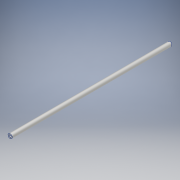
# Autodesk Inventor part: ScrewDriver
Saved by Autodesk Inventor 2017 (Build 210142000, 142)
## iProperties
Created: 2016-11-27
Part Number: ScrewDriver
Material: Aluminum 6061
Document SubType Name: Modeling
Designer: umr
Density: 2.7 g/cm^3
Appearance: Aluminum - Flat
Author: umr
Autodesk Inventor part; units mm, degrees
ref_plane "YZ Plane" through (0, 0, 0) normal (1, 0, 0) x (0, 1, 0)
ref_plane "XZ Plane" through (0, 0, 0) normal (0, 1, 0) x (-1, 0, 0)
sketch "Sketch1" plane through (0, 0, 0) normal (0, 1, 0) x (-1, 0, 0)
  circle A0 centre (0, 0) radius 8
  dimension "d0" = 16
  constraints: 1 centre point, 1 coincident
  measures "d0" diameter of A0
extrude "Extrusion1" add sketch "Sketch1" along normal blind 600
sketch "Sketch2" plane through (0, 0, 0) normal (0, -1, 0) x (1, 0, 0)
  circle A0 centre (0, 0) radius 3.5
  dimension "d7" = 7
  constraints: 1 centre point, 1 coincident
  measures "d7" diameter of A0
extrude "Extrusion2" cut sketch "Sketch2" against normal blind 10
ref_plane "Work Plane1" through (0, 300, 0) normal (0, -1, 0) x (1, 0, 0)
mirror "Mirror1" about plane through (0, 300, 0) normal (0, -1, 0) of "Extrusion2"
body "Solid1"
